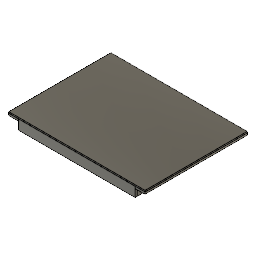
top (Autodesk Fusion 360 design; units mm, degrees)
Autodesk Fusion 360 part; units mm, degrees
sketch "Sketch1" plane through (0, 0, 0) normal (0, 0, 1) x (1, 0, 0) in component "A"
  line L0 (0, 0) -> (1219.2, 0)
  line L1 (1219.2, 0) -> (1219.2, 914.4)
  line L2 (1219.2, 914.4) -> (0, 914.4)
  line L3 (0, 914.4) -> (0, 0)
  dimension "d6" = 1219.2
  dimension "d7" = 914.4
  measures "d6" distance of L0.start
  measures "d7" distance of L0.start
extrude "Extrude1" add sketch "Sketch1" against normal blind 11.9062 makes body 1 in component "A"
sketch "Sketch1 (2)" plane through (0, 0, -11.9062) normal (0, 0, -1) x (1, 0, 0) in component "B"
  line L0 (0, 0) -> (0, -914.4)
  line L1 (0, -914.4) -> (1219.2, -914.4)
  line L2 (1219.2, -914.4) -> (1219.2, 0)
  line L3 (1219.2, 0) -> (0, 0)
  line L4 (0, 0) -> (88.9, 0)
  line L5 (88.9, 0) -> (88.9, -914.4)
  line L6 (88.9, -914.4) -> (0, -914.4)
  line L7 (0, -914.4) -> (0, 0)
  line L8 (609.6, 0) -> (609.6, -914.4) construction
  line L9 (1219.2, -914.4) -> (1219.2, 0)
  line L10 (1219.2, 0) -> (1130.3, 0)
  line L11 (1130.3, 0) -> (1130.3, -914.4)
  line L12 (1130.3, -914.4) -> (1219.2, -914.4)
  dimension "d10" = 914.4
  dimension "d11" = 88.9
  measures "d10" distance of L0.start
extrude "Extrude1'" add sketch "Sketch1 (2)" along normal blind 19.05 separate body contours L0 L1 L3 L4 L5 L6 L7 | L1 L2 L3 L9 L10 L11 L12 makes body 2 at (1159.9333, 304.8, -11.9062) makes body 3 at (59.2667, 609.6, -11.9062) in component "B"
sketch "Sketch1 (3)" plane through (0, 0, -11.9062) normal (0, 0, -1) x (1, 0, 0) in component "D"
  line L0 (0, 0) -> (0, -914.4)
  line L1 (0, -914.4) -> (1219.2, -914.4)
  line L2 (1219.2, -914.4) -> (1219.2, 0)
  line L3 (1219.2, 0) -> (0, 0)
  line L4 (88.9, 0) -> (1130.3, 0)
  line L5 (1130.3, 0) -> (1130.3, -19.05)
  line L6 (1130.3, -19.05) -> (88.9, -19.05)
  line L7 (88.9, -19.05) -> (88.9, 0)
  line L8 (0, -457.2) -> (1219.2, -457.2) construction
  line L9 (1130.3, -895.35) -> (88.9, -895.35)
  line L10 (88.9, -914.4) -> (1130.3, -914.4)
  line L11 (88.9, -895.35) -> (88.9, -914.4)
  line L12 (1130.3, -914.4) -> (1130.3, -895.35)
  dimension "d14" = 19.05
  dimension "d24" = 1041.4
  measures "d14" distance of L0.start
extrude "Extrude1''" add sketch "Sketch1 (3)" along normal blind 88.9 separate body contours L3 L4 L5 L6 L7 | L1 L9 L10 L11 L12 makes body 4 at (783.1667, 895.35, -41.5396) makes body 5 at (783.1667, 0, -41.5396) in component "D"
sketch "Sketch2" plane through (0, 0, -11.9062) normal (0, 0, -1) x (1, 0, 0) in component "C"
  line L0 (0, 0) -> (0, -914.4)
  line L1 (0, -914.4) -> (1219.2, -914.4)
  line L2 (1219.2, -914.4) -> (1219.2, 0)
  line L3 (1219.2, 0) -> (0, 0)
  line L4 (88.9, -19.05) -> (107.95, -19.05)
  line L5 (107.95, -19.05) -> (107.95, -895.35)
  line L6 (107.95, -895.35) -> (88.9, -895.35)
  line L7 (88.9, -895.35) -> (88.9, -19.05)
  line L8 (1130.3, -895.35) -> (88.9, -895.35)
  line L9 (600.075, -895.35) -> (600.075, -19.05)
  line L10 (619.125, -19.05) -> (619.125, -895.35)
  line L11 (619.125, -895.35) -> (600.075, -895.35)
  line L12 (600.075, -19.05) -> (619.125, -19.05)
  line L13 (1111.25, -895.35) -> (1111.25, -19.05)
  line L14 (1130.3, -19.05) -> (1130.3, -895.35)
  line L15 (1130.3, -895.35) -> (1111.25, -895.35)
  line L16 (1111.25, -19.05) -> (1130.3, -19.05)
  dimension "d17" = 19.05
  dimension "d20" = 1022.35
  dimension "d21" = 0
extrude "Extrude1'''" add sketch "Sketch2" along normal blind 88.9 separate body contours L4 L5 L6 L7 L8 | L8 L13 L14 L15 L16 | L8 L9 L10 L11 L12 makes body 6 at (1111.25, 603.25, -41.5396) makes body 7 at (600.075, 603.25, -41.5396) makes body 8 at (107.95, 311.15, -41.5396) in component "C"
component "A" placed x (1, 0, 0) y (0, 1, 0) z (0, 0, 1) at (0, 0, 0)
component "B" placed x (1, 0, 0) y (0, 1, 0) z (0, 0, 1) at (0, 0, 0)
component "C" placed x (1, 0, 0) y (0, 1, 0) z (0, 0, 1) at (0, 0, 0)
component "D" placed x (1, 0, 0) y (0, 1, 0) z (0, 0, 1) at (0, 0, 0)
equation "workbenchWidth = 36 in"
equation "workbenchLength = 48 in"
equation "plywoodThickness = ( 15 / 32 ) * 1 in"
equation "_1x = 0.75 in"
equation "x4 = 3.5 in"
equation "d6 = workbenchLength"
equation "d7 = workbenchWidth"
equation "d8 = -1 * plywoodThickness"
equation "d10 = workbenchWidth"
equation "d11 = x4"
equation "d12 = _1x"
equation "d14 = _1x"
equation "d15 = x4"
equation "d17 = _1x"
equation "d20 = workbenchLength - ( 2 * x4 ) - _1x"
equation "d22 = x4"
equation "d24 = workbenchLength - ( 2 * x4 )"
